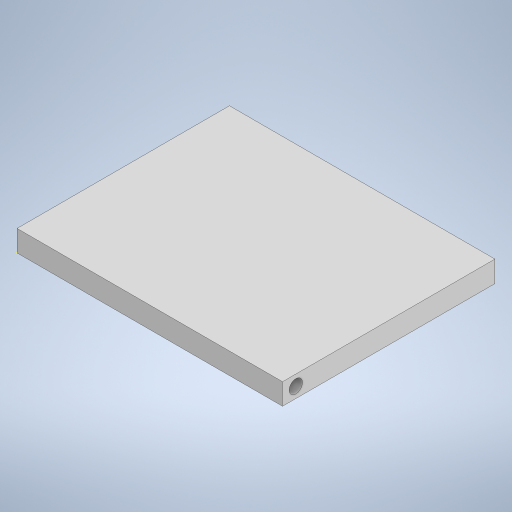
# Autodesk Inventor part: MoneyCase_Lid
Saved by Autodesk Inventor 2024 (Build 280153000, 153)
## iProperties
Created: 2025-03-28
Part Number: MoneyCase_Lid
Material: 一般
Document SubType Name: Modeling
Designer: TFG FabLab
Density: 1 g/cm^3
Appearance: 預設
Author: TFG FabLab
Autodesk Inventor part; units mm, degrees
ref_plane "YZ Plane" through (0, 0, 0) normal (1, 0, 0) x (0, 1, 0)
ref_plane "XZ Plane" through (0, 0, 0) normal (0, 1, 0) x (-1, 0, 0)
ref_plane "XY Plane" through (0, 0, 0) normal (0, 0, 1) x (1, 0, 0)
sketch "草圖1" plane through (0, 0, 0) normal (0, 1, 0) x (-1, 0, 0)
  line L0 (0, 0) -> (100, 0)
  line L1 (100, 0) -> (100, -80)
  line L2 (100, -80) -> (0, -80)
  line L3 (0, -80) -> (0, 0)
  dimension "d0" = 100
  dimension "d1" = 80
  constraints: 8 end point, 2 parallel, 1 horizontal, 1 perpendicular
  measures "d0" distance of L1.end L2.end
  measures "d1" distance of L0.end L1.end
extrude "擠出1" add sketch "草圖1" along normal blind 8
sketch "草圖2" plane through (0, 0, 0) normal (1, 0, 0) x (0, 0, -1)
  circle A0 centre (5, 4) radius 2.5
  line L0 (0, 0) -> (0, 8) projected
  line L1 (0, 8) -> (80, 8) projected
  point P0 (0, 4)
  dimension "d4" = 5
  dimension "d5" = 5
  dimension "d6" = 4
  constraints: 1 centre point, 1 midpoint
  measures "d4" diameter of A0
  measures "d5" distance of point (0, 4) A0.centre
  measures "d6" distance from line of L1 A0.centre
extrude "擠出2" cut sketch "草圖2" against normal blind 10
sketch "草圖3" plane through (-100, 0, -80) normal (-1, 0, 0) x (0, 0, 1)
  circle A0 centre (75, 4) radius 2.5 projected
  circle A1 centre (75, 4) radius 2.5
  point P0 (80, 0)
  constraints: 1 centre point, 1 coincident
extrude "擠出3" cut sketch "草圖3" against normal blind 10
sketch "草圖4" plane through (-100, 0, -80) normal (-1, 0, 0) x (0, 0, 1)
  point P0 (80, 0)
